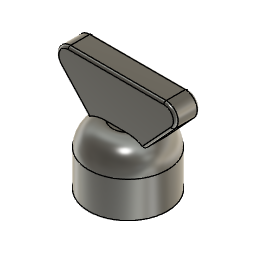
teigblume (Autodesk Fusion 360 design; units mm, degrees)
part number: 2025-04-22-12-01-25-163
part number: 2025-04-22-12-02-51-706
Autodesk Fusion 360 part; units mm, degrees
sketch "Skizze1" plane through (0, 0, 0) normal (0, 0, 1) x (1, 0, 0) in component "Teigblume"
  circle A0 centre (0, 0) radius 16.5
  dimension "d1" = 33
  constraint coincident A0.centre origin
  measures "d1" diameter of A0
extrude "Extrusion1" add sketch "Skizze1" along normal blind 25 in component "Teigblume"
fillet "Abrundung1" radius 10 1 edges at (-15.3834, -5.9667, 25) in component "Teigblume"
sketch "Skizze2" plane through (0, 0, 0) normal (0, 1, 0) x (1, 0, 0) in component "Teigblume"
  line L0 (6.5, -17) -> (31.5, -44)
  line L1 (31.5, -44) -> (-31.5, -44)
  line L2 (-31.5, -44) -> (-6.5, -17)
  line L3 (-6.5, -17) -> (6.5, -17)
  line L4 (-16.5, -15) -> (16.5, -15)
  dimension "d6" = 2
  dimension "d7" = 27
  dimension "d8" = 10
  dimension "d9" = 10
  dimension "d19" = 15
  dimension "d20" = 15
  constraint horizontal L1
  constraint parallel L1 L3
  measures "d6" distance of L0.start L4
  measures "d7" distance of L1 L3
  measures "d8" horizontal distance of L0.start L4.end
  measures "d9" horizontal distance of L2.end L4.start
  measures "d19" horizontal distance of L0.end L4.end
  measures "d20" horizontal distance of L1.end L4.start
extrude "Extrusion2" add sketch "Skizze2" along normal mid plane 10 in component "Teigblume"
fillet "Abrundung2" radius 5 2 edges at (-31.5, 0, 44) (31.5, 0, 44) in component "Teigblume"
fillet "Abrundung3" radius 1 10 edges at (-17.7705, 5, 29.1721) (-24.6379, 5, 41.0018) (0, 5, 44) (24.6379, 5, 41.0018) (17.7705, 5, 29.1721) (17.7705, -5, 29.1721) (24.6379, -5, 41.0018) (0, -5, 44) (-24.6379, -5, 41.0018) (-17.7705, -5, 29.1721) in component "Teigblume"
sketch "Skizze3" plane through (0, 0, 0) normal (0, 0, -1) x (1, 0, 0) in component "Teigblume"
  circle A0 centre (0, 0) radius 16.5
  line L0 (13.2791, 0) -> (6.6395, 11.5)
  line L1 (6.6395, 11.5) -> (-6.6395, 11.5)
  line L2 (-6.6395, 11.5) -> (-13.2791, 0)
  line L3 (-13.2791, 0) -> (-6.6395, -11.5)
  line L4 (-6.6395, -11.5) -> (6.6395, -11.5)
  line L5 (6.6395, -11.5) -> (13.2791, 0)
  dimension "d16" = 11.5
  constraint coincident A0.centre origin
  constraint horizontal L1
  measures "d16" distance of A0.centre L5
extrude "Extrusion3" cut sketch "Skizze3" against normal blind 13 contours L0 L1 L2 L3 L4 L5 in component "Teigblume"
component "Teigblume" placed x (1, 0, 0) y (0, 1, 0) z (0, 0, 1) at (0, 0, 0)
